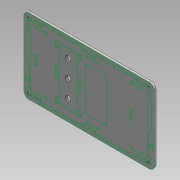
# Autodesk Inventor part: AK-C-C39-Bottom
Saved by Autodesk Inventor 2016 (Build 200138000, 138)
## iProperties
Created: 2016-06-05
Part Number: AK-C-C39-Bottom
Material: Generic
Document SubType Name: Modeling
Designer: admin
Density: 1 g/cm^3
Appearance: Default
Mass: 16.2918 g
Surface Area: 172.076 cm^2
Volume: 16.2918 cm^3
Author: admin
Autodesk Inventor part; units mm, degrees
ref_plane "YZ Plane" through (0, 0, 0) normal (1, 0, 0) x (0, 1, 0)
ref_plane "XZ Plane" through (0, 0, 0) normal (0, 1, 0) x (-1, 0, 0)
ref_plane "XY Plane" through (0, 0, 0) normal (0, 0, 1) x (1, 0, 0)
derived "AK-C-C39-Top.ipt"
sketch "Sketch1" plane through (0, 0, 0) normal (0, 1, 0) x (-1, 0, 0)
  arc A0 (55.5973, 28.6788) -> (54.2538, 30.0223) centre (55.5, 29.925) ccw
  arc A1 (-54.2538, 30.0223) -> (-55.5973, 28.6788) centre (-55.5, 29.925) ccw
  arc A2 (54.2538, -30.0223) -> (55.5973, -28.6788) centre (55.5, -29.925) ccw
  arc A3 (-55.5973, -28.6788) -> (-54.2538, -30.0223) centre (-55.5, -29.925) ccw
  line L0 (55.5, 34.425) -> (-55.5, 34.425)
  line L1 (55.5, -34.425) -> (-55.5, -34.425)
  line L2 (9.5866, 0) -> (-6.7847, 0) construction
  line L3 (0, -6.6233) -> (0, 6.4737) construction
  arc A4 (55.5, -34.425) -> (60, -29.925) centre (55.5, -29.925) ccw
  arc A5 (60, 29.925) -> (55.5, 34.425) centre (55.5, 29.925) ccw
  arc A6 (-55.5, 34.425) -> (-60, 29.925) centre (-55.5, 29.925) ccw
  arc A7 (-60, -29.925) -> (-55.5, -34.425) centre (-55.5, -29.925) ccw
  line L4 (57.5, 27.225) -> (57.5, 25.225)
  line L5 (57.5, 25.225) -> (55.5, 25.225)
  line L6 (55.5, 25.225) -> (55.5, 23.225)
  line L7 (55.5, 23.225) -> (57.5, 23.225)
  line L8 (57.5, 23.225) -> (57.5, 21.225)
  line L9 (57.5, 21.225) -> (55.5, 21.225)
  line L10 (55.5, 21.225) -> (55.5, 19.225)
  line L11 (55.5, 19.225) -> (57.8, 19.225)
  line L12 (57.8, 19.225) -> (57.8, -3.3607)
  line L13 (-57.5, 27.225) -> (-57.5, 25.225)
  line L14 (-57.5, 25.225) -> (-55.5, 25.225)
  line L15 (-55.5, 25.225) -> (-55.5, 23.225)
  line L16 (-55.5, 23.225) -> (-57.5, 23.225)
  line L17 (-57.5, 23.225) -> (-57.5, 21.225)
  line L18 (-57.5, 21.225) -> (-55.5, 21.225)
  line L19 (-55.5, 21.225) -> (-55.5, 19.225)
  line L20 (-55.5, 19.225) -> (-57.8, 19.225)
  line L21 (-57.8, 19.225) -> (-57.8, -3.3607)
  line L22 (57.5, 27.225) -> (55.3506, 27.225)
  line L23 (52.8, 29.7756) -> (52.8, 31.925)
  line L24 (52.8, 31.925) -> (50.8, 31.925)
  line L25 (50.8, 31.925) -> (50.8, 29.925)
  line L26 (50.8, 29.925) -> (48.8, 29.925)
  line L27 (48.8, 29.925) -> (48.8, 31.925)
  line L28 (48.8, 31.925) -> (46.8, 31.925)
  line L29 (46.8, 31.925) -> (46.8, 29.925)
  line L30 (46.8, 29.925) -> (44.8, 29.925)
  line L31 (44.8, 29.925) -> (44.8, 32.325)
  line L32 (44.8, 32.325) -> (5, 32.325)
  line L33 (5, 32.325) -> (5, 29.925)
  line L34 (5, 29.925) -> (3, 29.925)
  line L35 (3, 29.925) -> (3, 31.925)
  line L36 (3, 31.925) -> (1, 31.925)
  line L37 (1, 31.925) -> (1, 29.925)
  line L38 (1, 29.925) -> (-1, 29.925)
  line L39 (-1, 29.925) -> (-1, 31.925)
  line L40 (-1, 31.925) -> (-3, 31.925)
  line L41 (-3, 31.925) -> (-3, 29.925)
  line L42 (-3, 29.925) -> (-5, 29.925)
  line L43 (-5, 29.925) -> (-5, 32.325)
  line L44 (-5, 32.325) -> (-44.8, 32.325)
  line L45 (-44.8, 32.325) -> (-44.8, 29.925)
  line L46 (-44.8, 29.925) -> (-46.8, 29.925)
  line L47 (-46.8, 29.925) -> (-46.8, 31.925)
  line L48 (-46.8, 31.925) -> (-48.8, 31.925)
  line L49 (-48.8, 31.925) -> (-48.8, 29.925)
  line L50 (-48.8, 29.925) -> (-50.8, 29.925)
  line L51 (-50.8, 29.925) -> (-50.8, 31.925)
  line L52 (-50.8, 31.925) -> (-52.8, 31.925)
  line L53 (-52.8, 31.925) -> (-52.8, 29.7756)
  line L54 (-55.3506, 27.225) -> (-57.5, 27.225)
  line L55 (55.5973, 28.6788) -> (54.9971, 28.0786)
  line L56 (54.2538, 30.0223) -> (53.6536, 29.4221)
  line L57 (55.5, 29.925) -> (51.9091, 26.3341) construction
  arc A8 (52.8, 29.7756) -> (53.6536, 29.4221) centre (53.3, 29.7756) ccw
  arc A9 (54.9971, 28.0786) -> (55.3506, 27.225) centre (55.3506, 27.725) ccw
  line L58 (-55.5973, 28.6788) -> (-54.9971, 28.0786)
  line L59 (-54.2538, 30.0223) -> (-53.6536, 29.4221)
  arc A10 (-53.6536, 29.4221) -> (-52.8, 29.7756) centre (-53.3, 29.7756) ccw
  arc A11 (-55.3506, 27.225) -> (-54.9971, 28.0786) centre (-55.3506, 27.725) ccw
  line L60 (57.8, -3.3607) -> (55, -7.6074)
  line L61 (55, -7.6074) -> (55, -16.775)
  arc A12 (56.5, -18.525) -> (58.5, -18.525) centre (57.5, -19.275) ccw
  line L62 (58.5, -18.525) -> (58.5, -16.775)
  line L63 (56.5, -18.525) -> (56.5, -16.775)
  line L64 (55, -16.775) -> (56.5, -16.775)
  line L65 (58.5, -16.775) -> (60, -16.775)
  line L66 (57.5, -16.4962) -> (57.5, -11.7384) construction
  line L67 (-57.8, -3.3607) -> (-55, -7.6074)
  line L68 (-55, -7.6074) -> (-55, -16.775)
  arc A13 (-56.5, -15.025) -> (-58.5, -15.025) centre (-57.5, -14.275) ccw
  line L69 (-58.5, -15.025) -> (-58.5, -16.775)
  line L70 (-56.5, -15.025) -> (-56.5, -16.775)
  line L71 (-55, -16.775) -> (-56.5, -16.775)
  line L72 (-58.5, -16.775) -> (-60, -16.775)
  line L73 (-57.5, -20.9142) -> (-57.5, -16.6435) construction
  line L74 (44.8, -32.325) -> (5, -32.325)
  line L75 (5, -32.325) -> (5, -29.925)
  line L76 (5, -29.925) -> (3, -29.925)
  line L77 (3, -29.925) -> (3, -31.925)
  line L78 (3, -31.925) -> (1, -31.925)
  line L79 (1, -31.925) -> (1, -29.925)
  line L80 (1, -29.925) -> (-1, -29.925)
  line L81 (-1, -29.925) -> (-1, -31.925)
  line L82 (-1, -31.925) -> (-3, -31.925)
  line L83 (-3, -31.925) -> (-3, -29.925)
  line L84 (-3, -29.925) -> (-5, -29.925)
  line L85 (-5, -29.925) -> (-5, -32.325)
  line L86 (-5, -32.325) -> (-44.8, -32.325)
  line L87 (55, -17.425) -> (55, -25.225)
  line L88 (55, -25.225) -> (57.5, -25.225)
  line L89 (57.5, -25.225) -> (57.5, -27.225)
  line L90 (57.5, -27.225) -> (55.3506, -27.225)
  line L91 (52.8, -29.7756) -> (52.8, -31.925)
  line L92 (52.8, -31.925) -> (50.8, -31.925)
  line L93 (50.8, -31.925) -> (50.8, -29.925)
  line L94 (50.8, -29.925) -> (48.8, -29.925)
  line L95 (48.8, -29.925) -> (48.8, -31.925)
  line L96 (48.8, -31.925) -> (46.8, -31.925)
  line L97 (46.8, -31.925) -> (46.8, -29.925)
  line L98 (46.8, -29.925) -> (44.8, -29.925)
  line L99 (44.8, -29.925) -> (44.8, -32.325)
  line L100 (-44.8, -32.325) -> (-44.8, -29.925)
  line L101 (-44.8, -29.925) -> (-46.8, -29.925)
  line L102 (-46.8, -29.925) -> (-46.8, -31.925)
  line L103 (-46.8, -31.925) -> (-48.8, -31.925)
  line L104 (-48.8, -31.925) -> (-48.8, -29.925)
  line L105 (-48.8, -29.925) -> (-50.8, -29.925)
  line L106 (-50.8, -29.925) -> (-50.8, -31.925)
  line L107 (-50.8, -31.925) -> (-52.8, -31.925)
  line L108 (-52.8, -31.925) -> (-52.8, -29.7756)
  line L109 (-55.3506, -27.225) -> (-57.5, -27.225)
  line L110 (-57.5, -27.225) -> (-57.5, -25.225)
  line L111 (-57.5, -25.225) -> (-55, -25.225)
  line L112 (-55, -25.225) -> (-55, -17.425)
  line L113 (54.9971, -28.0786) -> (55.5973, -28.6788)
  line L114 (53.6536, -29.4221) -> (54.2538, -30.0223)
  arc A14 (55.3506, -27.225) -> (54.9971, -28.0786) centre (55.3506, -27.725) ccw
  arc A15 (53.6536, -29.4221) -> (52.8, -29.7756) centre (53.3, -29.7756) ccw
  line L115 (-54.2538, -30.0223) -> (-53.6536, -29.4221)
  line L116 (-55.5973, -28.6788) -> (-54.9971, -28.0786)
  arc A16 (-52.8, -29.7756) -> (-53.6536, -29.4221) centre (-53.3, -29.7756) ccw
  arc A17 (-54.9971, -28.0786) -> (-55.3506, -27.225) centre (-55.3506, -27.725) ccw
  line L117 (55, -17.425) -> (56.5, -17.425)
  line L118 (58.5, -17.425) -> (60, -17.425)
  line L119 (60, -29.925) -> (60, -17.425)
  line L120 (60, -16.775) -> (60, 29.925)
  line L121 (-55, -17.425) -> (-56.5, -17.425)
  line L122 (-56.5, -17.425) -> (-56.5, -16.775)
  line L123 (-58.5, -16.775) -> (-58.5, -17.425)
  line L124 (-58.5, -17.425) -> (-60, -17.425)
  line L125 (-60, -29.925) -> (-60, -17.425)
  line L126 (-60, -16.775) -> (-60, 29.925)
  point P0 (0, 0)
sketch "Sketch2" plane through (0, 0, 0) normal (0, 1, 0) x (-1, 0, 0)
  line L0 (27.75, 22.5) -> (27.75, -22.5)
  arc A0 (38.75, -27) -> (40.5, -27) centre (39.625, -27) ccw
  arc A1 (40.5, -25.25) -> (38.75, -25.25) centre (39.625, -25.25) ccw
  arc A2 (38.75, 25.25) -> (40.25, 25.25) centre (39.5, 25.25) ccw
  line L1 (48.75, -27) -> (40.5, -27)
  line L2 (38.75, -27) -> (38.75, -25.25)
  line L3 (40.5, -25.25) -> (48.75, -25.25)
  line L4 (1.75, -27) -> (-8.25, -27)
  line L5 (-8.25, -25.25) -> (1.75, -25.25)
  line L6 (-40, -27) -> (-48.25, -27)
  line L7 (-48.25, -25.25) -> (-40, -25.25)
  line L8 (-48.25, 25.25) -> (-40, 25.25)
  line L9 (-40, 27) -> (-48.25, 27)
  line L10 (1.75, 25.25) -> (-8.25, 25.25)
  line L11 (-8.25, 27) -> (1.75, 27)
  line L12 (48.75, 25.25) -> (40.25, 25.25)
  line L13 (38.75, 25.25) -> (38.75, 27)
  line L14 (40.25, 27) -> (48.75, 27)
  line L15 (-39.5, -4) -> (-37.75, -4)
  arc A3 (-37.75, -4) -> (-37.75, -2.5) centre (-37.75, -3.25) ccw
  arc A4 (-39.5, -2.5) -> (-39.5, -4) centre (-39.5, -3.25) ccw
  arc A5 (-37.75, 2.5) -> (-37.75, 4) centre (-37.75, 3.25) ccw
  arc A6 (-39.5, 4) -> (-39.5, 2.5) centre (-39.5, 3.25) ccw
  line L16 (-37.75, -2.5) -> (-37.75, 2.5)
  line L17 (-39.5, 4) -> (-37.75, 4)
  line L18 (-39.5, 2.5) -> (-39.5, -2.5)
  arc A7 (40.25, 27) -> (38.75, 27) centre (39.5, 27) ccw
  line L19 (48.25, -2.5) -> (48.25, 2.5)
  line L20 (50, -2.5) -> (50, 2.5)
  line L21 (50, -4) -> (48.25, -4)
  line L22 (50, 4) -> (48.25, 4)
  arc A8 (50, -4) -> (50, -2.5) centre (50, -3.25) ccw
  arc A9 (48.25, -2.5) -> (48.25, -4) centre (48.25, -3.25) ccw
  arc A10 (50, 2.5) -> (50, 4) centre (50, 3.25) ccw
  arc A11 (48.25, 4) -> (48.25, 2.5) centre (48.25, 3.25) ccw
  line L23 (55, -25.225) -> (-54.9956, -25.225) construction
  line L24 (55.5, 25.225) -> (55.5, 23.225)
  line L25 (57.5, 25.225) -> (55.5, 25.225)
  arc A12 (10.75, -22.5) -> (12.75, -24.5) centre (12.75, -22.5) ccw
  arc A13 (25.75, -24.5) -> (27.75, -22.5) centre (25.75, -22.5) ccw
  arc A14 (12.75, 24.5) -> (10.75, 22.5) centre (12.75, 22.5) ccw
  arc A15 (27.75, 22.5) -> (25.75, 24.5) centre (25.75, 22.5) ccw
  line L26 (19.25, -23.7063) -> (19.25, 24.6931) construction
  line L27 (-57.5, 25.225) -> (-55.5, 25.225)
  line L28 (-55.5, 25.225) -> (-55.5, 23.225)
  line L29 (-57.5, -25.225) -> (-55, -25.225)
  line L30 (-55, -25.225) -> (-55, -17.425)
  line L31 (55, -25.225) -> (57.5, -25.225)
  line L32 (55.5, 25.225) -> (-55.5, 25.225) construction
  line L33 (25.75, -24.5) -> (12.75, -24.5)
  line L34 (12.75, 24.5) -> (25.75, 24.5)
  line L35 (3.3524, -20) -> (-16.6476, -20)
  line L36 (-16.6476, -20) -> (-16.6476, 20)
  line L37 (-16.6476, 20) -> (3.3524, 20)
  line L38 (3.3524, 20) -> (3.3524, -20)
  line L39 (-23.9878, -15) -> (-31.9878, -15) construction
  line L40 (-31.9878, -15) -> (-31.9878, -7) construction
  line L41 (-31.9878, -7) -> (-23.9878, -7) construction
  line L42 (-23.9878, -7) -> (-23.9878, -15) construction
  line L43 (-34.9878, -15) -> (-42.9878, -15) construction
  line L44 (-42.9878, -15) -> (-42.9878, -7) construction
  line L45 (-42.9878, -7) -> (-34.9878, -7) construction
  line L46 (-34.9878, -7) -> (-34.9878, -15) construction
  line L47 (-23.9878, -4) -> (-31.9878, -4) construction
  line L48 (-31.9878, -4) -> (-31.9878, 4) construction
  line L49 (-31.9878, 4) -> (-23.9878, 4) construction
  line L50 (-23.9878, 4) -> (-23.9878, -4) construction
  line L51 (-34.9878, -4) -> (-42.9878, -4) construction
  line L52 (-42.9878, -4) -> (-42.9878, 4) construction
  line L53 (-42.9878, 4) -> (-34.9878, 4) construction
  line L54 (-34.9878, 4) -> (-34.9878, -4) construction
  line L55 (-23.9878, 7) -> (-31.9878, 7) construction
  line L56 (-31.9878, 7) -> (-31.9878, 15) construction
  line L57 (-31.9878, 15) -> (-23.9878, 15) construction
  line L58 (-23.9878, 15) -> (-23.9878, 7) construction
  line L59 (-34.9878, 7) -> (-42.9878, 7) construction
  line L60 (-42.9878, 7) -> (-42.9878, 15) construction
  line L61 (-42.9878, 15) -> (-34.9878, 15) construction
  line L62 (-34.9878, 15) -> (-34.9878, 7) construction
  line L63 (25.75, -22.5) -> (12.75, -22.5) construction
  line L64 (12.75, -22.5) -> (12.75, -9.5) construction
  line L65 (12.75, -9.5) -> (25.75, -9.5) construction
  line L66 (25.75, -9.5) -> (25.75, -22.5) construction
  line L67 (25.75, -6.5) -> (12.75, -6.5) construction
  line L68 (12.75, -6.5) -> (12.75, 6.5) construction
  line L69 (12.75, 6.5) -> (25.75, 6.5) construction
  line L70 (25.75, 6.5) -> (25.75, -6.5) construction
  line L71 (25.75, 9.5) -> (12.75, 9.5) construction
  line L72 (12.75, 9.5) -> (12.75, 22.5) construction
  line L73 (12.75, 22.5) -> (25.75, 22.5) construction
  line L74 (25.75, 22.5) -> (25.75, 9.5) construction
  line L75 (31.9633, -16) -> (17.7262, -16) construction
  line L76 (31.9633, 16) -> (18.8213, 16) construction
  line L77 (0, -6.6233) -> (0, 6.4737) construction
  line L78 (9.5866, 0) -> (-6.7847, 0) construction
  line L79 (57.8, 19.225) -> (57.8, -3.3607)
  line L80 (57.8, -3.3607) -> (55, -7.6074)
  line L81 (55.5, 19.225) -> (57.8, 19.225)
  line L82 (55.5, 29.925) -> (51.9091, 26.3341) construction
  line L83 (51.25, -29) -> (44.125, -29)
  line L84 (43.25, -29.875) -> (43.25, -31)
  line L85 (43.25, -31) -> (6.5, -31)
  line L86 (6.5, -31) -> (6.5, -29.875)
  line L87 (5.625, -29) -> (-5.625, -29)
  line L88 (-6.5, -29.875) -> (-6.5, -31)
  line L89 (-6.5, -31) -> (-43.25, -31)
  line L90 (-43.25, -31) -> (-43.25, -29.875)
  line L91 (-44.125, -29) -> (-51.25, -29)
  line L92 (-51.25, -29) -> (-53.75, -26.5)
  line L93 (-53.75, -26.5) -> (-53.75, 26.5)
  line L94 (-53.75, 26.5) -> (-51.25, 29)
  line L95 (-51.25, 29) -> (-44.125, 29)
  line L96 (-43.25, 29.875) -> (-43.25, 31)
  line L97 (-43.25, 31) -> (-6.5, 31)
  line L98 (-6.5, 31) -> (-6.5, 29.875)
  line L99 (-5.625, 29) -> (5.625, 29)
  line L100 (6.5, 29.875) -> (6.5, 31)
  line L101 (43.25, 31) -> (43.25, 29.875)
  line L102 (43.25, 31) -> (6.5, 31)
  line L103 (44.125, 29) -> (51.25, 29)
  line L104 (51.25, 29) -> (53.75, 26.5)
  line L105 (53.75, 26.5) -> (53.75, -26.5)
  line L106 (53.75, -26.5) -> (51.25, -29)
  line L107 (44.8, -32.325) -> (5, -32.325)
  line L108 (5, -32.325) -> (5, -29.925)
  line L109 (5, -29.925) -> (3, -29.925)
  line L110 (44.8, -29.925) -> (44.8, -32.325)
  line L111 (46.8, -29.925) -> (44.8, -29.925)
  line L112 (52.8, -29.7756) -> (52.8, -31.925)
  arc A16 (53.6536, -29.4221) -> (52.8, -29.7756) centre (53.3, -29.7756) ccw
  arc A17 (55.3506, -27.225) -> (54.9971, -28.0786) centre (55.3506, -27.725) ccw
  line L113 (55, -17.425) -> (55, -25.225)
  line L114 (-34.9878, 7) -> (-42.9878, 15) construction
  line L115 (-31.9878, 7) -> (-23.9878, 15) construction
  line L116 (-31.9878, -7) -> (-23.9878, -15) construction
  line L117 (-34.9878, -7) -> (-42.9878, -15) construction
  arc A18 (3.3524, 19) -> (2.3524, 20) centre (2.3524, 19) ccw
  arc A19 (-15.6476, 20) -> (-16.6476, 19) centre (-15.6476, 19) ccw
  arc A20 (2.3524, -20) -> (3.3524, -19) centre (2.3524, -19) ccw
  arc A21 (-16.6476, -19) -> (-15.6476, -20) centre (-15.6476, -19) ccw
  line L118 (10.75, 7.999) -> (10.75, 8)
  line L119 (10.75, -22.5) -> (10.75, 22.5)
  arc A22 (7.5, 20) -> (9.25, 20) centre (8.375, 20) ccw
  arc A23 (9.25, 23.5) -> (9.25, 25) centre (9.25, 24.25) ccw
  arc A24 (7.5, 25) -> (7.5, 23.5) centre (7.5, 24.25) ccw
  line L120 (9.25, 25) -> (7.5, 25)
  line L121 (7.5, 23.5) -> (7.5, 20)
  line L122 (9.25, 20) -> (9.25, 23.5)
  line L123 (7.5, -20) -> (7.5, -23.25)
  line L124 (7.5, -25) -> (9.25, -25)
  line L125 (9.25, -23.25) -> (9.25, -20)
  arc A25 (9.25, -20) -> (7.5, -20) centre (8.375, -20) ccw
  arc A26 (9.25, -25) -> (9.25, -23.25) centre (9.25, -24.125) ccw
  arc A27 (7.5, -23.25) -> (7.5, -25) centre (7.5, -24.125) ccw
  arc A28 (31, -25) -> (31, -23.25) centre (31, -24.125) ccw
  arc A29 (29.25, -23.25) -> (29.25, -25) centre (29.25, -24.125) ccw
  arc A30 (31, -20) -> (29.25, -20) centre (30.125, -20) ccw
  arc A31 (29.25, 25) -> (29.25, 23.5) centre (29.25, 24.25) ccw
  arc A32 (29.25, 20) -> (31, 20) centre (30.125, 20) ccw
  line L126 (29.25, -20) -> (29.25, -23.25)
  line L127 (29.25, -25) -> (31, -25)
  line L128 (31, -23.25) -> (31, -20)
  line L129 (31, 25) -> (29.25, 25)
  line L130 (31, 23.5) -> (31, 20)
  line L131 (29.25, 20) -> (29.25, 23.5)
  arc A33 (31, 23.5) -> (31, 25) centre (31, 24.25) ccw
  arc A34 (-48.25, -25.25) -> (-48.25, -27) centre (-48.25, -26.125) ccw
  arc A35 (-8.25, -25.25) -> (-8.25, -27) centre (-8.25, -26.125) ccw
  arc A36 (48.75, -27) -> (48.75, -25.25) centre (48.75, -26.125) ccw
  arc A37 (-48.25, 27) -> (-48.25, 25.25) centre (-48.25, 26.125) ccw
  arc A38 (48.75, 25.25) -> (48.75, 27) centre (48.75, 26.125) ccw
  arc A39 (-8.25, 27) -> (-8.25, 25.25) centre (-8.25, 26.125) ccw
  arc A40 (44.125, -29) -> (43.25, -29.875) centre (44.125, -29.875) ccw
  arc A41 (6.5, -29.875) -> (5.625, -29) centre (5.625, -29.875) ccw
  arc A42 (-5.625, -29) -> (-6.5, -29.875) centre (-5.625, -29.875) ccw
  arc A43 (-43.25, -29.875) -> (-44.125, -29) centre (-44.125, -29.875) ccw
  arc A44 (-44.125, 29) -> (-43.25, 29.875) centre (-44.125, 29.875) ccw
  arc A45 (-6.5, 29.875) -> (-5.625, 29) centre (-5.625, 29.875) ccw
  arc A46 (5.625, 29) -> (6.5, 29.875) centre (5.625, 29.875) ccw
  arc A47 (43.25, 29.875) -> (44.125, 29) centre (44.125, 29.875) ccw
  line L132 (29.25, 4) -> (29.25, -4)
  line L133 (31, -4) -> (31, 4)
  line L134 (7.5, 4) -> (7.5, -4)
  line L135 (9.25, -4) -> (9.25, 4)
  arc A48 (31, 4) -> (29.25, 4) centre (30.125, 4) ccw
  arc A49 (29.25, -4) -> (31, -4) centre (30.125, -4) ccw
  arc A50 (9.25, 4) -> (7.5, 4) centre (8.375, 4) ccw
  arc A51 (7.5, -4) -> (9.25, -4) centre (8.375, -4) ccw
  line L136 (-14.75, 30.3253) -> (-31.75, 30.3253) construction
  line L137 (-31.75, 30.3253) -> (-31.75, 22.4164) construction
  line L138 (-31.75, 22.4164) -> (-14.75, 22.4164) construction
  line L139 (-14.75, 22.4164) -> (-14.75, 30.3253) construction
  line L140 (-23.25, 29.9722) -> (-23.25, 20.9797) construction
  line L141 (57.5, 27.225) -> (57.5, 25.225)
  line L142 (-57.5, 27.225) -> (-57.5, 25.225)
  arc A52 (-38.25, 27) -> (-40, 27) centre (-39.125, 27) ccw
  arc A53 (-40, 25.25) -> (-38.25, 25.25) centre (-39.125, 25.25) ccw
  line L143 (-38.25, 27) -> (-38.25, 25.25)
  arc A54 (-38.25, -25.25) -> (-40, -25.25) centre (-39.125, -25.25) ccw
  arc A55 (-40, -27) -> (-38.25, -27) centre (-39.125, -27) ccw
  line L144 (-38.25, -25.25) -> (-38.25, -27)
  arc A56 (1.75, 25.25) -> (1.75, 27) centre (1.75, 26.125) ccw
  arc A57 (1.75, -27) -> (1.75, -25.25) centre (1.75, -26.125) ccw
  line L145 (-60, -16.775) -> (-60, 29.925)
  point P0 (10.75, 0)
  point P1 (27.75, 0)
  point P2 (19.25, -22.5)
  point P3 (19.25, -24.5)
  point P4 (25.75, -16)
  point P5 (25.75, 16)
  point P6 (53.75, -25.225)
  point P7 (-53.75, -25.225)
  point P8 (-23.25, 18)
  point P9 (-23.25, -18)
  point P10 (-23.25, 30.3253)
sketch "Sketch5" plane through (0, 0, 0) normal (0, 1, 0) x (-1, 0, 0)
  line L0 (60, -16.775) -> (60, 29.925) projected
  line L1 (60, -29.925) -> (60, -17.425) projected
  line L2 (60, -16.775) -> (60, -17.425)
  line L3 (-60, -16.775) -> (-60, 29.925) projected
  line L4 (-60, -29.925) -> (-60, -17.425) projected
  line L5 (-60, -16.775) -> (-60, -17.425)
  arc A0 (60, 29.925) -> (55.5, 34.425) centre (55.5, 29.925) ccw projected
  line L6 (55.5, 34.425) -> (-55.5, 34.425) projected
  arc A1 (-55.5, 34.425) -> (-60, 29.925) centre (-55.5, 29.925) ccw projected
  arc A2 (-60, -29.925) -> (-55.5, -34.425) centre (-55.5, -29.925) ccw projected
  line L7 (55.5, -34.425) -> (-55.5, -34.425) projected
  arc A3 (55.5, -34.425) -> (60, -29.925) centre (55.5, -29.925) ccw projected
  point P0 (0, 0)
  constraints: 4 end point, 2 vertical
extrude "Extrusion1" add sketch "Sketch5" along normal blind 2
sketch "Sketch6" plane through (0, 2, 0) normal (0, 1, 0) x (1, 0, 0)
  point P0 (0, 0)
  point P1 (-55.5, -29.925)
  point P2 (55.5, -29.925)
  point P3 (55.5, 29.925)
  point P4 (-55.5, 29.925)
hole "Hole1" at (-55.5, 2, -29.925) at (55.5, 2, -29.925) at (55.5, 2, 29.925) at (-55.5, 2, 29.925) direction (0, -1, 0) diameter 3 end through all countersink diameter 5 countersink angle 90
sketch "Sketch7" plane through (0, 2, 0) normal (0, 1, 0) x (1, 0, 0)
  line L0 (-19.25, 23.7063) -> (-19.25, -24.6931) construction
  line L1 (-31.9633, -16) -> (-18.8213, -16) construction
  line L2 (-9.5866, 0) -> (6.7847, 0) construction
  line L3 (-31.9633, 16) -> (-17.7262, 16) construction
  point P0 (0, 0)
  point P1 (-19.25, 16)
  point P2 (-19.25, 0)
  point P3 (-19.25, -16)
  constraints: 6 point on line
hole "Hole2" at (-19.25, 2, -16) at (-19.25, 2, 0) at (-19.25, 2, 16) direction (0, -1, 0) diameter 5 end through all
body "Solid2"
